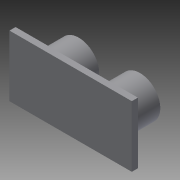
# Autodesk Inventor part: ultrason
Saved by Autodesk Inventor 2014 SP1 (Build 180222100, 222)
## iProperties
Created: 2015-02-03
Part Number: ultrason
Material: Générique
Document SubType Name: Modeling
Designer: astralien3000
Density: 1 g/cm^3
Appearance: Par défaut
Author: astralien3000
Autodesk Inventor part; units mm, degrees
ref_plane "YZ Plane" through (0, 0, 0) normal (1, 0, 0) x (0, 1, 0)
ref_plane "XZ Plane" through (0, 0, 0) normal (0, 1, 0) x (-1, 0, 0)
ref_plane "XY Plane" through (0, 0, 0) normal (0, 0, 1) x (1, 0, 0)
sketch "Esquisse1" plane through (0, 0, 0) normal (0, 1, 0) x (-1, 0, 0)
  line L0 (-15, 7.5) -> (15, 7.5)
  line L1 (15, 7.5) -> (15, -7.5)
  line L2 (15, -7.5) -> (-15, -7.5)
  line L3 (-15, -7.5) -> (-15, 7.5)
  point P0 (0, 0)
  dimension "d0" = 15
  dimension "d1" = 30
  dimension "d2" = 15
  dimension "d3" = 7.5
  constraints: 8 end point, 2 parallel, 1 horizontal, 1 perpendicular
  measures "d0" distance of L2.end L0.start
  measures "d1" distance of L0.start L0.end
  measures "d2" distance from line of point (0, 0) L1
  measures "d3" distance from line of point (0, 0) L0
extrude "Extrusion1" add sketch "Esquisse1" along normal blind 1.5
sketch "Esquisse2" plane through (0, 1.5, 0) normal (0, 1, 0) x (1, 0, 0)
  circle A0 centre (-7.5, 0) radius 5
  circle A1 centre (7.5, 0) radius 5
  point P0 (0, 0)
  dimension "d6" = 10
  dimension "d7" = 10
  dimension "d8" = 15
  dimension "d9" = 7.5
  constraints: 2 centre point
  measures "d6" diameter of A0
  measures "d7" diameter of A1
  measures "d8" distance of A1.centre A0.centre
  measures "d9" distance of point (0, 0) A1.centre
extrude "Extrusion2" add sketch "Esquisse2" along normal blind 8
equation "\"d2\" = 0.5 * d1"
equation "\"d3\" = 0.5 * d0"
equation "\"d7\" = d6"
equation "\"d9\" = 0.5 * d8"
